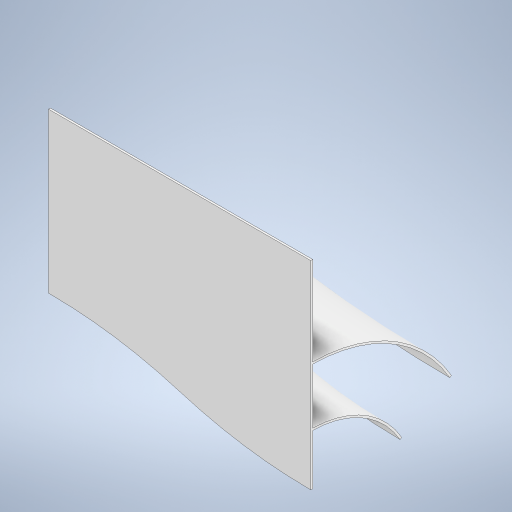
# Autodesk Inventor part: Diffusoren mit Trennwand
Saved by Autodesk Inventor 2023 (Build 270158000, 158)
## iProperties
Created: 2022-02-28
Part Number: Diffusoren mit Trennwand
Material: Generisch
Document SubType Name: Modeling
Designer: Marcel
Density: 1 g/cm^3
Appearance: Weiß
Author: Marcel
Autodesk Inventor part; units mm, degrees
ref_plane "YZ Plane" through (0, 0, 0) normal (1, 0, 0) x (0, 1, 0)
ref_plane "XZ Plane" through (0, 0, 0) normal (0, 1, 0) x (-1, 0, 0)
ref_plane "XY Plane" through (0, 0, 0) normal (0, 0, 1) x (1, 0, 0)
sketch "Skizze1" plane through (0, 0, 0) normal (0, 0, 1) x (1, 0, 0)
  line L0 (0, 0) -> (200, 0) construction
  line L1 (200, 0) -> (200, 40.1) construction
  line L2 (200, 40.1) -> (200, 41.6)
  line L3 (0, 0) -> (0, 70) construction
  line L4 (0, 70) -> (0, 71.5)
  arc A0 (100, 55.05) -> (0, 70) centre (0, -271.9232) ccw
  arc A1 (100, 55.05) -> (200, 40.1) centre (200, 382.0232) ccw
  arc A2 (100, 56.55) -> (0, 71.5) centre (0, -270.4232) ccw
  arc A3 (100, 56.55) -> (200, 41.6) centre (200, 383.5232) ccw
  line L5 (0, 71.5) -> (0, 101.5) construction
  line L6 (200, 41.6) -> (200, 78.6) construction
  line L7 (0, 101.5) -> (0, 103)
  line L8 (200, 78.6) -> (200, 80.1)
  line L9 (0, 103) -> (0, 133) construction
  line L10 (0, 133) -> (0, 134.5)
  line L11 (200, 80.1) -> (200, 122.4) construction
  line L12 (200, 122.4) -> (200, 123.9)
  arc A4 (100, 90.05) -> (200, 78.6) centre (200, 521.0062) ccw
  arc A5 (100, 91.55) -> (200, 80.1) centre (200, 522.5062) ccw
  arc A6 (100, 90.05) -> (0, 101.5) centre (0, -340.9062) ccw
  arc A7 (100, 91.55) -> (0, 103) centre (0, -339.4062) ccw
  arc A8 (100, 129.2) -> (200, 123.9) centre (200, 1069.9462) ccw
  arc A9 (100, 127.7) -> (0, 133) centre (0, -813.0462) ccw
  arc A10 (100, 127.7) -> (200, 122.4) centre (200, 1068.4462) ccw
  arc A11 (100, 129.2) -> (0, 134.5) centre (0, -811.5462) ccw
  line L13 (0, 0) -> (0, 190) construction
  line L14 (0, 190) -> (200, 190) construction
  line L15 (200, 190) -> (200, 191.5) construction
  line L16 (0, 190) -> (0, 191.5) construction
  line L17 (0, 191.5) -> (200, 191.5) construction
  line L18 (0, 0) -> (200, 0)
  point P0 (143.9749, 47.5506)
  point P1 (136.2206, 124.2462)
  point P2 (104.2284, 54.3303)
  dimension "d0" = 200
  dimension "d1" = 40.1
  dimension "d2" = 1.5
  dimension "d3" = 70
  dimension "d4" = 1.5
  dimension "d5" = 30
  dimension "d6" = 37
  dimension "d7" = 1.5
  dimension "d8" = 1.5
  dimension "d9" = 30
  dimension "d10" = 1.5
  dimension "d11" = 42.3
  dimension "d12" = 1.5
  dimension "d13" = 100
  dimension "d14" = 100
  dimension "d15" = 100
  dimension "d56" = 190
  dimension "d57" = 200
  dimension "d58" = 90
  dimension "d59" = 1.5
  dimension "d60" = 1.5
  dimension "d61" = 200
  dimension "d89" = 55.5
  constraints: 38 end point, 24 point on circle, 12 centre point, 9 equal radius, 9 line through centre, 9 vertical, 4 point on line, 4 vertical alignment, 3 perpendicular, 2 horizontal, 1 coincident
  measures "d0" distance of L0.start L0.end
  measures "d1" distance of L0.end L1.end
  measures "d2" distance of L1.end L2.end
  measures "d3" distance of L0.start L3.end
  measures "d4" distance of L3.end L4.end
  measures "d5" distance of L4.end L5.end
  measures "d6" distance of L2.end L6.end
  measures "d7" distance of L5.end L7.end
  measures "d8" distance of L6.end L8.end
  measures "d9" distance of L7.end L9.end
  measures "d10" distance of L9.end L10.end
  measures "d11" distance of L8.end L11.end
  measures "d12" distance of L11.end L12.end
  measures "d13" distance from line of L3 A0.start
  measures "d14" distance from line of L5 A4.start
  measures "d15" distance from line of L9 A9.start
  measures "d56" distance of L13.start L13.end
  measures "d57" distance of L13.end L14.end
  measures "d58" angle of L13 L14
  measures "d59" distance of L14.end L15.end
  measures "d60" distance of L13.end L16.end
  measures "d61" distance of L13.start L18.end
  measures "d89" distance of L13.end L10.end
revolve "Umdrehung1" add sketch "Skizze1" angle 60 about axis through (0, 0, 0) along (-1, 0, 0) contours L7 A7 A5 L8 A4 A6 | L10 A11 A8 L12 A10 A9
sketch "Skizze3" plane through (0, 0, 0) normal (0, 0, 1) x (1, 0, 0)
  line L0 (200, 175.0528) -> (200, 191.5)
  line L1 (0, 191.5) -> (200, 191.5)
  arc A0 (100, 55.05) -> (0, 70) centre (0, -271.9232) ccw projected
  arc A1 (100, 55.05) -> (200, 40.1) centre (200, 382.0232) ccw projected
  line L2 (0, 70) -> (0, 191.5)
  line L3 (200, 191.5) -> (200, 40.1)
  point P0 (0, 0)
  point P1 (0, 0)
  point P2 (0, 0)
  point P3 (143.9749, 47.5506)
  point P4 (136.2206, 124.2462)
  point P5 (104.2284, 54.3303)
  point P6 (0, 0)
  dimension "d90" = 191.5
  dimension "d91" = 200
  constraints: 8 end point, 2 coincident, 2 vertical, 1 perpendicular
  measures "d90" distance from line of L1 point (0, 0)
  measures "d91" distance of L1.start L0.end
extrude "Extrusion1" add sketch "Skizze3" against normal blind 1.5
